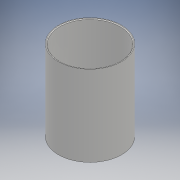
# Autodesk Inventor part: A0003
Saved by Autodesk Inventor 2017 (Build 210142000, 142)
## iProperties
Part Number: A0003
Material: 一般
Document SubType Name: Modeling
Designer: lygfy
Density: 1 g/cm^3
Appearance: 預設
Author: lygfy
Autodesk Inventor part; units mm, degrees
ref_plane "YZ Plane" through (0, 0, 0) normal (1, 0, 0) x (0, 1, 0)
ref_plane "XZ Plane" through (0, 0, 0) normal (0, 1, 0) x (-1, 0, 0)
ref_plane "XY Plane" through (0, 0, 0) normal (0, 0, 1) x (1, 0, 0)
sketch "草圖1" plane through (0, 0, 0) normal (1, 0, 0) x (0, 1, 0)
  line L0 (23.5, 30) -> (23, 30)
  line L1 (22.5, 29.5) -> (22.5, -29.5)
  line L2 (23, -30) -> (23.5, -30)
  line L3 (23.5, -30) -> (23.5, 30)
  line L4 (0, -42) -> (0, 42) construction
  line L5 (22.5, 29.5) -> (23, 30)
  line L6 (22.5, -29.5) -> (23, -30)
  point P0 (0, 0)
  point P1 (22.5, -30)
  point P2 (22.5, 30)
  point P3 (22.5, 0)
  dimension "d0" = 45
  dimension "d1" = 1
  dimension "d2" = 0.5
  dimension "d3" = 0.5
  dimension "d4" = 0.5
  dimension "d5" = 0.5
  dimension "d6" = 60
  constraints: 12 end point, 4 point on line, 2 parallel, 1 horizontal, 1 horizontal alignment, 1 midpoint, 1 perpendicular
  measures "d0" diameter of L1 L4
  measures "d1" distance of point (22.5, -30) L2.end
  measures "d2" distance of L1.start point (22.5, 30)
  measures "d3" distance of L0.end point (22.5, 30)
  measures "d4" distance of L1.end point (22.5, -30)
  measures "d5" distance of L2.start point (22.5, -30)
  measures "d6" distance of L2.end L0.start
revolve "迴轉1" add sketch "草圖1" angle 360 about axis through (0, 0, -10) along (0, 0, 1)
equation "\"d3\" = d2"
equation "\"d4\" = d2"
equation "\"d5\" = d4"
